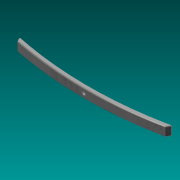
# Autodesk Inventor part: leaf 4
Saved by Autodesk Inventor 2014 SP2 (Build 180246200, 246)
## iProperties
Created: 2019-07-17
Part Number: leaf 4
Material: Steel, Carbon
Document SubType Name: Modeling
Designer: USER PC
Density: 7.87 g/cm^3
Appearance: Semi-Polished
Mass: 1735.35 g
Surface Area: 436.624 cm^2
Volume: 220.501 cm^3
Author: USER PC
Autodesk Inventor part; units mm, degrees
ref_plane "YZ Plane" through (0, 0, 0) normal (1, 0, 0) x (0, 1, 0)
ref_plane "XZ Plane" through (0, 0, 0) normal (0, 1, 0) x (-1, 0, 0)
ref_plane "XY Plane" through (0, 0, 0) normal (0, 0, 1) x (1, 0, 0)
sketch "Sketch1" plane through (0, 0, 0) normal (0, 0, 1) x (1, 0, 0)
  arc A0 (0.1634, -106.6592) -> (254.828, -79.7002) centre (0.1634, 1109.6463) ccw
  arc A1 (0.1634, -121.6592) -> (244.7719, -97.118) centre (0.1634, 1109.6463) ccw
  line L0 (254.828, -79.7002) -> (244.7719, -97.118)
  line L1 (254.828, -79.7002) -> (274.9404, -79.7002) construction
  line L2 (0.1634, -121.6592) -> (0.1634, -88.4091)
  arc A2 (-244.445, -97.118) -> (0.1634, -121.6592) centre (0.1634, 1109.6463) ccw
  arc A3 (-254.5012, -79.7002) -> (0.1634, -106.6592) centre (0.1634, 1109.6463) ccw
  line L3 (-254.5012, -79.7002) -> (-244.445, -97.118)
  point P0 (0, 0)
  point P1 (226.5563, -100.6675)
  dimension "d0" = 15
  dimension "d1" = 120
  constraints: 9 point on circle, 8 end point, 4 centre point, 2 symmetric about line, 1 equal length, 1 horizontal, 1 perpendicular, 2 other
  measures "d0" radial gap between concentric circles of A1 A0
  measures "d1" angle of L0 L1
extrude "Extrusion1" add sketch "Sketch1" along normal blind 30
fillet "Fillet1" radius 3 12 edges at (-127.8803, -99.9007, 30) (123.0817, -115.5086, 30) (128.2072, -99.9007, 0) (249.8, -88.4091, 30) (254.828, -79.7002, 15) (244.7719, -97.118, 15) (249.8, -88.4091, 0) (123.0817, -115.5086, 0) (-249.4731, -88.4091, 0) (-244.445, -97.118, 15) (-249.4731, -88.4091, 30) (-254.5012, -79.7002, 15)
sketch "Sketch2" plane through (0, 0, 0) normal (0, 1, 0) x (-1, 0, 0)
  line L0 (0, 0) -> (0, 15)
  circle A0 centre (0, 15) radius 5
  dimension "d5" = 15
  dimension "d6" = 10
  constraints: 2 end point, 1 centre point, 1 coincident, 1 vertical
  measures "d5" distance of L0.start L0.end
  measures "d6" diameter of A0
extrude "Extrusion2" cut sketch "Sketch2" against normal blind 300
body "Solid1"
